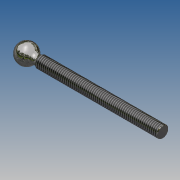
# Autodesk Inventor part: M6x60
Saved by Autodesk Inventor 2015 (Build 190159000, 159)
## iProperties
Created: 2015-01-09
Part Number: M6x60
Material: Stahl, hochfest, niedrig legiert
Document SubType Name: Modeling
Designer: Marc
Density: 7.85 g/cm^3
Appearance: Stahl - poliert
Mass: 18.5141 g
Surface Area: 15.5615 cm^2
Volume: 2.35848 cm^3
Author: Marc
Autodesk Inventor part; units mm, degrees
ref_plane "YZ Plane" through (0, 0, 0) normal (1, 0, 0) x (0, 1, 0)
ref_plane "XZ Plane" through (0, 0, 0) normal (0, 1, 0) x (-1, 0, 0)
ref_plane "XY Plane" through (0, 0, 0) normal (0, 0, 1) x (1, 0, 0)
sketch "Skizze1" plane through (0, 0, 0) normal (0, 0, 1) x (1, 0, 0)
  line L0 (0, -0.6) -> (0, 3.6) projected
  line L1 (-31.5, 0) -> (31.5, 0)
  line L2 (31.5, 0) -> (31.5, 3)
  line L3 (31.5, 3) -> (-31.5, 3)
  line L4 (-31.5, 3) -> (-31.5, 0)
  dimension "d2" = 63
  dimension "d3" = 3
  constraints: 8 end point, 2 parallel, 1 horizontal, 1 perpendicular, 1 other
  measures "d2" distance of L3.end L2.end
  measures "d3" distance of L2.end L1.end
revolve "Umdrehung1" add sketch "Skizze1" angle 360 about axis through (-31.5, 0, 0) along (1, 0, 0)
thread "Gewinde1" size "M6x1" class "6g" standard "ANSI Metric M Profile" full length
chamfer "Fase1" distance 0.3 angle 45 1 edges at (31.5, -3, 0)
sketch "Skizze2" plane through (0, 0, 0) normal (0, 0, 1) x (1, 0, 0)
  line L0 (-31.5, -3) -> (-31.5, 3) projected
  line L1 (31.2, -3) -> (31.2, 3) projected
  line L2 (-58.1911, 0) -> (44.3485, 0) projected
  line L3 (0, -4.8487) -> (0, 8.0921) projected
  arc A0 (-34.9614, 3) -> (-43.9614, 0) centre (-38.9614, 0) ccw
  arc A1 (-34.9614, 3) -> (-31.5, 3) centre (-33.2307, 4.7589) ccw
  line L4 (-31.5, -3) -> (-31.5, 3) projected
  line L5 (-43.9614, 0) -> (-31.5, 0)
  line L6 (-31.5, 3) -> (-31.5, 0)
  point P0 (0, 0)
  dimension "d10" = 5
  constraints: 4 end point, 4 point on circle, 2 centre point, 1 collinear, 1 midpoint
  measures "d10" radius of A0
revolve "Umdrehung2" add sketch "Skizze2" angle 360 about axis through (-43.9614, 0, 0) along (1, 0, 0)
